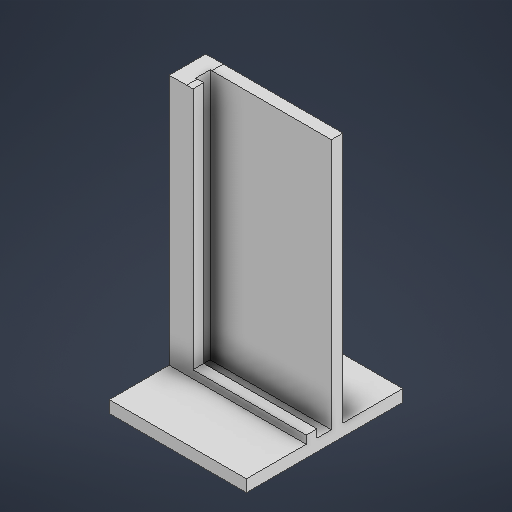
# Autodesk Inventor part: КРЕПЛ НОМЕРА
Saved by Autodesk Inventor 2025 (Build 290162000, 162)
## iProperties
Created: 2024-11-26
Part Number: КРЕПЛ НОМЕРА
Material: Типовые
Document SubType Name: Modeling
Designer: Phantom
Density: 1 g/cm^3
Appearance: По умолчанию
Author: Phantom
Autodesk Inventor part; units mm, degrees
ref_plane "YZ Plane" through (0, 0, 0) normal (1, 0, 0) x (0, 1, 0)
ref_plane "XZ Plane" through (0, 0, 0) normal (0, 1, 0) x (-1, 0, 0)
ref_plane "XY Plane" through (0, 0, 0) normal (0, 0, 1) x (1, 0, 0)
sketch "Эскиз1" plane through (0, 0, 0) normal (0, 0, 1) x (1, 0, 0)
  line L0 (0, 0) -> (194, 0)
  line L1 (194, 0) -> (194, 63)
  line L2 (194, 63) -> (0, 63)
  line L3 (0, 63) -> (0, 0)
  dimension "d0" = 194
  dimension "d1" = 63
  constraints: 8 end point, 2 parallel, 1 horizontal, 1 perpendicular
  measures "d0" distance of L2.end L1.end
  measures "d1" distance of L1.end L0.end
extrude "Выдавливание1" add sketch "Эскиз1" along normal blind 3.2
sketch "Эскиз2" plane through (0, 0, 0) normal (0, 0, -1) x (-1, 0, 0)
  line L0 (-97, 63) -> (-97, -37)
  line L1 (0, 0) -> (-2, 0)
  line L2 (4.3861, 62.9632) -> (4.3861, 0)
  line L3 (4.3861, 0) -> (0, 0)
  line L4 (4.3861, 62.9632) -> (-1.6137, 63)
  line L5 (-1.6137, 63) -> (-1.6137, 0)
  line L6 (-194, 0) -> (-192, 0)
  line L7 (-198.3861, 62.9632) -> (-198.3861, 0)
  line L8 (-198.3861, 0) -> (-194, 0)
  line L9 (-198.3861, 62.9632) -> (-192.3863, 63)
  line L10 (-192.3863, 63) -> (-192.3863, 0)
  dimension "d19" = 6
  constraints: 22 end point, 6 symmetric about line, 4 point on line, 1 vertical
  measures "d19" distance of L2.start L4.end
extrude "Выдавливание2" add sketch "Эскиз2" against normal blind 9.2
sketch "Эскиз4" plane through (0, 0, 3.2) normal (0, 0, 1) x (1, 0, 0)
  line L0 (0, 63) -> (0, 62.9901) projected
  line L1 (0, 62.9901) -> (30, 62.9901)
  line L2 (194, 63) -> (0, 63) projected
  line L3 (0, 62.9901) -> (30, 62.9901) construction
  line L4 (30, 62.9901) -> (30, -44)
  line L5 (0, 62.9901) -> (30, 62.9901)
  line L6 (30, 62.9901) -> (30, -60)
  line L7 (30, -60) -> (0, -60)
  line L8 (0, -60) -> (0, 62.9901)
  line L9 (97, 63) -> (97, -80)
  line L10 (194, 63) -> (194, 62.9901)
  line L11 (194, 62.9901) -> (164, 62.9901)
  line L12 (194, 62.9901) -> (164, 62.9901) construction
  line L13 (164, 62.9901) -> (164, -44)
  line L14 (194, 62.9901) -> (164, 62.9901)
  line L15 (164, 62.9901) -> (164, -60)
  line L16 (164, -60) -> (194, -60)
  line L17 (194, -60) -> (194, 62.9901)
  line L18 (194, 63) -> (192.3863, 63) projected
  line L19 (0, 63) -> (0, 62.9901) projected
  line L20 (1.6137, 0) -> (192.3863, 0) projected
  line L21 (194, 62.9901) -> (194, 63) projected
  line L22 (0, 62.9901) -> (1.6137, 63) projected
  line L23 (1.6137, 63) -> (0, 63) projected
  line L24 (1.6137, 63) -> (1.6137, 0) projected
  line L25 (192.3863, 0) -> (192.3863, 63) projected
  line L26 (192.3863, 63) -> (1.6137, 63) projected
  line L27 (192.3863, 63) -> (194, 62.9901) projected
  point P0 (0, 0)
  point P1 (194, 0)
  point P2 (30, 0)
  point P3 (164, 0)
  constraints: 32 end point, 8 symmetric about line, 3 parallel, 2 horizontal, 2 perpendicular, 1 collinear, 1 midpoint, 1 vertical
extrude "Выдавливание4" cut sketch "Эскиз4" against normal through all contours L2 L22 L0 | L22 L24 L1 | L2 L9 L20 L4 L1 L24 | L2 L25 L11 L13 L20 L9 | L27 L11 L25 | L2 L10 L27
sketch "Эскиз5" plane through (0, 0, 9.2) normal (0, 0, 1) x (1, 0, 0)
  line L0 (2, 0) -> (1.6137, 63) projected
  line L1 (2, 0) -> (1.9877, 2)
  line L2 (192.3863, 63) -> (192, 0) projected
  line L3 (1.9877, 2) -> (192, 2)
  line L4 (192, 2) -> (192, 0)
  line L5 (192, 0) -> (1.9877, 0)
  line L6 (1.9877, 0) -> (1.9877, 2)
  line L7 (30, 62.9901) -> (30, 0) projected
  line L8 (30, 62.9901) -> (164, 62.9901)
  line L9 (164, 62.9901) -> (164, -48)
  line L10 (164, -48) -> (30, -48)
  line L11 (30, -48) -> (30, 62.9901)
  line L12 (1.9877, 2) -> (1.6137, 2)
  line L13 (1.6137, 0) -> (1.6137, 63) projected
  line L14 (1.9877, 0) -> (1.6137, 0)
  line L15 (192, 2) -> (192.0123, 2)
  line L16 (192.0123, 2) -> (192, 0)
  line L17 (192, 0) -> (192, 0)
  line L18 (192, 0) -> (192, 0)
  line L19 (192.0123, 2) -> (192.3863, 2)
  line L20 (192.3863, 2) -> (192.3863, 0)
  line L21 (192.3863, 0) -> (192, 0)
  point P0 (0, 0)
  point P1 (164, 2)
  point P2 (164, 0)
  point P3 (30, 2)
  dimension "d16" = 2
  constraints: 36 end point, 7 perpendicular, 4 horizontal, 4 parallel, 4 point on line, 1 collinear
  measures "d16" distance of L0.start L1.end
sketch "Эскиз6" plane through (0, 62.9901, 3.2) normal (0, 1, 0) x (1, 0, 0)
  line L0 (30, 0) -> (1.6137, 0) projected
  line L1 (1.6137, 0) -> (-0.3863, 0)
  line L2 (-0.3863, 0) -> (-0.3863, -3)
  line L3 (-0.3863, -3) -> (1.6137, -3)
  line L4 (1.6137, -3) -> (1.6137, 0)
  line L5 (192.3863, 0) -> (194.3863, 0)
  line L6 (194.3863, 0) -> (194.3863, -3)
  line L7 (194.3863, -3) -> (192.3863, -3)
  line L8 (192.3863, -3) -> (192.3863, 0)
  point P0 (0, 3.2)
  dimension "d20" = 2
  dimension "d21" = 2
  constraints: 16 end point, 4 parallel, 2 horizontal, 2 perpendicular, 1 point on line
  measures "d20" distance of L3.end L2.end
  measures "d21" distance of L6.end L7.end
extrude "Выдавливание6" cut sketch "Эскиз6" against normal through all
sketch "Эскиз7" plane through (0, 62.9901, 0) normal (0, 1, 0) x (1, 0, 0)
  line L0 (-40, 32) -> (232, 32)
  line L1 (232, 32) -> (232, -40)
  line L2 (232, -40) -> (-40, -40)
  line L3 (-40, -40) -> (-40, 32)
  point P0 (0, 0)
  constraints: 8 end point, 2 parallel, 1 horizontal, 1 perpendicular
extrude "Выдавливание7" cut sketch "Эскиз7" along normal blind 10
extrude "Выдавливание8" add sketch "Эскиз5" against normal up to surface (3 mm away) contours L5 L6 L0 | L0 L3 L7 L5 | L6 L14 L13 L12 | L7 L3 L9 L5 | L9 L3 L4 L5 | L2 L19 L20 L21
sketch "Эскиз8" plane through (0, 0, 9.2) normal (0, 0, 1) x (1, 0, 0)
  line L0 (30, 0) -> (30, 62.9901) projected
  line L1 (30, 62.9901) -> (164, 62.9901)
  line L2 (164, 62.9901) -> (164, -18)
  line L3 (164, -18) -> (30, -18)
  line L4 (30, -18) -> (30, 62.9901)
  point P0 (0, 0)
  constraints: 8 end point, 2 parallel, 1 horizontal, 1 perpendicular
extrude "Выдавливание9" cut sketch "Эскиз8" against normal through all
sketch "Эскиз9" plane through (192, 0, 6.2) normal (-0.9999812, 0.0061309, 0) x (0, 0, 1)
  line L0 (0, 0) -> (0, 2) projected
  line L1 (3, 0) -> (0, 0) projected
  line L2 (3, 2) -> (3, 0) projected
  line L3 (3, 2) -> (0, 2) projected
  point P0 (-6.2, -1.1771)
extrude "Выдавливание10" add sketch "Эскиз9" along normal up to surface surface through (192, 2, 9.2) normal (1, 0, 0)
sketch "Эскиз10" plane through (198.3861, 0, 0) normal (0, -1, 0) x (1, 0, 0)
  line L0 (-168.3861, 6.2) -> (-168.3861, 9.2) projected
  line L1 (-202.7723, 9.2) -> (-168.3861, 9.2) projected
  line L2 (-202.7723, 0) -> (-202.7723, 9.2) projected
  line L3 (-168.3861, 0) -> (-202.7723, 0) projected
  line L4 (-168.3861, 0) -> (-168.3861, 3.2) projected
  line L5 (-198.7724, 3.2) -> (-168.3861, 3.2) projected
  line L6 (-198.7724, 3.2) -> (-198.7724, 6.2) projected
  line L7 (-168.3861, 6.2) -> (-198.7724, 6.2) projected
  line L8 (-3.9999, 6.2) -> (-34.3861, 6.2) projected
  line L9 (-3.9999, 6.2) -> (-3.9999, 3.2) projected
  line L10 (-34.3861, 3.2) -> (-3.9999, 3.2) projected
  line L11 (-34.3861, 3.2) -> (-34.3861, 0) projected
  line L12 (0, 0) -> (-34.3861, 0) projected
  line L13 (0, 0) -> (0, 9.2) projected
  line L14 (-34.3861, 9.2) -> (0, 9.2) projected
  line L15 (-34.3861, 9.2) -> (-34.3861, 6.2) projected
  line L16 (-168.3861, 6.2) -> (-168.3861, 3.2)
  line L17 (-34.3861, 6.2) -> (-34.3861, 3.2)
  point P0 (-198.3861, 0)
  constraints: 4 end point, 1 parallel, 1 vertical
extrude "Выдавливание11" add sketch "Эскиз10" along normal blind 3
sketch "Эскиз11" plane through (198.3861, -3, 0) normal (0, -1, 0) x (1, 0, 0)
  line L0 (-198.3861, 9.2) -> (-202.7723, 9.2) projected
  line L1 (-202.7723, 9.2) -> (-202.7723, 24.2)
  line L2 (-168.3861, 9.2) -> (-196.7724, 9.2) projected
  line L3 (-202.7723, 24.2) -> (-168.3861, 24.2)
  line L4 (-168.3861, 24.2) -> (-168.3861, 9.2)
  line L5 (-168.3861, 9.2) -> (-202.7723, 9.2)
  line L6 (-202.7723, 9.2) -> (-202.7723, 24.2)
  line L7 (-168.3861, 0) -> (-202.7723, 0)
  line L8 (-202.7723, 0) -> (-202.7723, -15)
  line L9 (-202.7723, -15) -> (-168.3861, -15)
  line L10 (-168.3861, -15) -> (-168.3861, 0)
  line L11 (0, 9.2) -> (-4.3861, 9.2) projected
  line L12 (0, 9.2) -> (0, 24.2)
  line L13 (-6.3861, 9.2) -> (-34.3861, 9.2) projected
  line L14 (0, 24.2) -> (-34.3861, 24.2)
  line L15 (-34.3861, 24.2) -> (-34.3861, 9.2)
  line L16 (-34.3861, 9.2) -> (0, 9.2)
  line L17 (0, 9.2) -> (0, 24.2)
  line L18 (-34.3861, 0) -> (-4.3861, 0) projected
  line L19 (-34.3861, 0) -> (0, 0)
  line L20 (0, 0) -> (0, -15)
  line L21 (0, -15) -> (-34.3861, -15)
  line L22 (-34.3861, -15) -> (-34.3861, 0)
  point P0 (-198.3861, 0)
  dimension "d34" = 15
  dimension "d35" = 15
  constraints: 36 end point, 8 parallel, 4 horizontal, 4 perpendicular, 3 point on line, 2 vertical
  measures "d34" distance of L0.end L1.end
  measures "d35" distance of L11.start L12.end
extrude "Выдавливание12" add sketch "Эскиз11" against normal up to surface (3 mm away)
sketch "Эскиз12" plane through (164, -3, 24.2) normal (0, 0, 1) x (1, 0, 0)
  line L0 (-47, 132) -> (117, 132)
  line L1 (117, 132) -> (117, -136)
  line L2 (117, -136) -> (-47, -136)
  line L3 (-47, -136) -> (-47, 132)
  point P0 (-164, 3)
  constraints: 8 end point, 2 parallel, 1 horizontal, 1 perpendicular
extrude "Выдавливание13" cut sketch "Эскиз12" against normal through all
sketch "Эскиз13" plane through (0, 62.9901, 3.2) normal (0, 1, 0) x (1, 0, 0)
  line L0 (-0.3863, -3) -> (-0.3863, 0) projected
  line L1 (-0.3863, -1.5) -> (-0.3863, 0.3)
  line L2 (-0.3863, 0.3) -> (-0.3863, -3.3)
  line L3 (-0.3863, 0.3) -> (49.6137, 0.3)
  line L4 (49.6137, 0.3) -> (49.6137, -3.3)
  line L5 (49.6137, -3.3) -> (-0.3863, -3.3)
  line L6 (-0.3863, -3.3) -> (-0.3863, 0.3)
  point P0 (0, 3.2)
  point P1 (-0.3863, -3.3)
  dimension "d40" = 1.8
  dimension "d41" = 3.6
  dimension "d42" = 50
  dimension "d43" = 3.6
  constraints: 12 end point, 2 parallel, 1 collinear, 1 horizontal, 1 midpoint, 1 perpendicular, 1 point on line
  measures "d40" distance of L1.start L1.end
  measures "d41" distance of L1.end L2.end
  measures "d42" distance of L4.end L5.end
  measures "d43" distance of L3.end L4.end
extrude "Выдавливание14" cut sketch "Эскиз13" against normal up to surface (62.9901 mm away)
